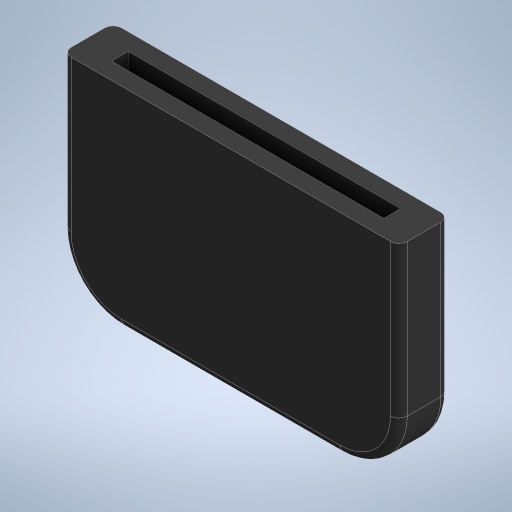
# Autodesk Inventor part: Door Stop Bumper
Saved by Autodesk Inventor 2024 (Build 280153000, 153)
## iProperties
Created: 2024-11-27
Part Number: Door Stop Bumper
Material: Rubber
Document SubType Name: Modeling
Designer: Ishaan
Density: 0.93 g/cm^3
Appearance: Rubber - Black
Author: Ishaan
Autodesk Inventor part; units mm, degrees
ref_plane "YZ Plane" through (0, 0, 0) normal (1, 0, 0) x (0, 1, 0)
ref_plane "XZ Plane" through (0, 0, 0) normal (0, 1, 0) x (-1, 0, 0)
ref_plane "XY Plane" through (0, 0, 0) normal (0, 0, 1) x (1, 0, 0)
sketch "Sketch3" plane through (0, 0, 0) normal (0, 0, 1) x (1, 0, 0)
  line L0 (16, -10.5) -> (-16, -10.5)
  line L1 (-16, -10.5) -> (-16, 10.5)
  line L2 (-16, 10.5) -> (16, 10.5)
  line L3 (16, 10.5) -> (16, -10.5)
  line L4 (16, -10.5) -> (-16, 10.5) construction
  line L5 (-16, -10.5) -> (16, 10.5) construction
  circle A0 centre (0, -1.5) radius 3.5
  line L6 (-2.5, -3.9495) -> (2.5, -3.9495)
  line L7 (2.5, -3.9495) -> (2.5, -10.5)
  line L8 (2.5, -10.5) -> (-2.5, -10.5)
  line L9 (-2.5, -10.5) -> (-2.5, -3.9495)
  point P0 (0, 0)
  dimension "d24" = 32
  dimension "d25" = 21
  dimension "d26" = 7
  dimension "d27" = 9
  dimension "d28" = 5
  constraints: 20 end point, 4 parallel, 2 horizontal, 2 midpoint, 2 perpendicular, 2 point on circle, 1 centre point, 1 point on line, 1 vertical alignment
  measures "d24" distance of L1.end L2.end
  measures "d25" distance of L0.end L1.end
  measures "d26" diameter of A0
  measures "d27" distance from line of A0.centre L0
  measures "d28" distance between parallel lines of L7 L9
extrude "Extrusion5" add sketch "Sketch3" along normal mid plane 1.6 contours L0 L7 A0 L9 L1 L2 L3
fillet "Fillet2" radius 1 2 edges at (-2.5, -3.9495, 0) (2.5, -3.9495, 0)
fillet "Fillet3" radius 3 2 edges at (-16, -10.5, 0) (16, -10.5, 0)
fillet "Fillet4" radius 1 2 edges at (-2.5, -10.5, 0) (2.5, -10.5, 0)
sketch "Sketch4" plane through (0, 0, 0) normal (0, 0, 1) x (1, 0, 0)
  arc A0 (2.7222, -3.6999) -> (2.5, -4.3284) centre (3.5, -4.3284) ccw projected
  arc A1 (2.7222, -3.6999) -> (-2.7222, -3.6999) centre (0, -1.5) ccw projected
  arc A2 (-2.5, -4.3284) -> (-2.7222, -3.6999) centre (-3.5, -4.3284) ccw projected
  line L0 (-2.5, -4.3284) -> (-2.5, -9.5) projected
  arc A3 (-3.5, -10.5) -> (-2.5, -9.5) centre (-3.5, -9.5) ccw projected
  line L1 (-3.5, -10.5) -> (-13, -10.5) projected
  arc A4 (-16, -7.5) -> (-13, -10.5) centre (-13, -7.5) ccw projected
  line L2 (-16, -7.5) -> (-16, 10.5) projected
  line L3 (-16, 10.5) -> (16, 10.5) projected
  line L4 (16, 10.5) -> (16, -7.5) projected
  arc A5 (13, -10.5) -> (16, -7.5) centre (13, -7.5) ccw projected
  line L5 (13, -10.5) -> (3.5, -10.5) projected
  arc A6 (2.5, -9.5) -> (3.5, -10.5) centre (3.5, -9.5) ccw projected
  line L6 (2.5, -9.5) -> (2.5, -4.3284) projected
  line L7 (-16.2, 10.7) -> (-16.2, -7.5)
  arc A7 (-16.2, -7.5) -> (-13, -10.7) centre (-13, -7.5) ccw
  line L8 (-13, -10.7) -> (-3.5, -10.7)
  arc A8 (-3.5, -10.7) -> (-2.3, -9.5) centre (-3.5, -9.5) ccw
  line L9 (-2.3, -9.5) -> (-2.3, -4.3284)
  arc A9 (-2.3, -4.3284) -> (-2.5667, -3.5742) centre (-3.5, -4.3284) ccw
  arc A10 (2.5667, -3.5742) -> (-2.5667, -3.5742) centre (0, -1.5) ccw
  arc A11 (2.5667, -3.5742) -> (2.3, -4.3284) centre (3.5, -4.3284) ccw
  line L10 (2.3, -4.3284) -> (2.3, -9.5)
  arc A12 (2.3, -9.5) -> (3.5, -10.7) centre (3.5, -9.5) ccw
  line L11 (3.5, -10.7) -> (13, -10.7)
  arc A13 (13, -10.7) -> (16.2, -7.5) centre (13, -7.5) ccw
  line L12 (16.2, -7.5) -> (16.2, 10.7)
  line L13 (16.2, 10.7) -> (-16.2, 10.7)
  line L14 (-20, 14.5) -> (-20, -7.5)
  arc A14 (-20, -7.5) -> (-13, -14.5) centre (-13, -7.5) ccw
  line L15 (-13, -14.5) -> (13, -14.5)
  arc A15 (13, -14.5) -> (20, -7.5) centre (13, -7.5) ccw
  line L16 (20, -7.5) -> (20, 14.5)
  line L17 (20, 14.5) -> (-20, 14.5)
  line L18 (-20, 10.5) -> (20, 10.5)
  point P0 (0, 0)
  point P1 (-16.2, 10.5)
  point P2 (16.2, 10.5)
  dimension "d34" = 0.2
  dimension "d35" = 4
  constraints: 24 end point, 18 point on circle, 9 centre point, 2 point on line, 1 collinear, 1 perpendicular, 1 tangent, 17 other
  measures "d34" distance between parallel lines of L2 L7
  measures "d35" distance between parallel lines of L2 L14
extrude "Extrusion6" add sketch "Sketch4" along normal mid plane 2 separate body contours L18 L16 A15 L15 A14 L14 L7 A7 L8 A8 L9 A9 A10 A11 L10 A12 L11 A13 L12
sketch "Sketch5" plane through (0, 0, 1) normal (0, 0, 1) x (1, 0, 0)
  line L0 (-16.2, -7.5) -> (-16.2, 10.5) projected
  line L1 (-16.2, 10.5) -> (-20, 10.5) projected
  line L2 (-20, 10.5) -> (-20, -7.5) projected
  arc A0 (-20, -7.5) -> (-13, -14.5) centre (-13, -7.5) ccw projected
  line L3 (-13, -14.5) -> (13, -14.5) projected
  arc A1 (13, -14.5) -> (20, -7.5) centre (13, -7.5) ccw projected
  line L4 (20, -7.5) -> (20, 10.5) projected
  line L5 (20, 10.5) -> (16.2, 10.5) projected
  line L6 (16.2, 10.5) -> (16.2, -7.5) projected
  arc A2 (13, -10.7) -> (16.2, -7.5) centre (13, -7.5) ccw projected
  line L7 (13, -10.7) -> (3.5, -10.7) projected
  arc A3 (2.3, -9.5) -> (3.5, -10.7) centre (3.5, -9.5) ccw projected
  line L8 (2.3, -9.5) -> (2.3, -4.3284) projected
  arc A4 (2.5667, -3.5742) -> (2.3, -4.3284) centre (3.5, -4.3284) ccw projected
  arc A5 (2.5667, -3.5742) -> (-2.5667, -3.5742) centre (0, -1.5) ccw projected
  arc A6 (-2.3, -4.3284) -> (-2.5667, -3.5742) centre (-3.5, -4.3284) ccw projected
  line L9 (-2.3, -4.3284) -> (-2.3, -9.5) projected
  arc A7 (-3.5, -10.7) -> (-2.3, -9.5) centre (-3.5, -9.5) ccw projected
  line L10 (-3.5, -10.7) -> (-13, -10.7) projected
  arc A8 (-16.2, -7.5) -> (-13, -10.7) centre (-13, -7.5) ccw projected
  line L11 (-16.2, 10.5) -> (16.2, 10.5)
  point P0 (0, 0)
  constraints: 2 end point, 1 horizontal
extrude "Extrusion7" add sketch "Sketch5" along normal blind 2
mirror "Mirror1" about plane through (0, 0, 0) normal (0, 0, 1) of "Extrusion7"
fillet "Fillet5" radius 1 10 edges at (20, 1.5, -3) (0, -14.5, -3) (-17.9497, -12.4497, -3) (-20, 1.5, -3) (17.9497, -12.4497, -3) (20, 1.5, 3) (0, -14.5, 3) (-17.9497, -12.4497, 3) (-20, 1.5, 3) (17.9497, -12.4497, 3)
body "Solid1"
body "Solid3"
